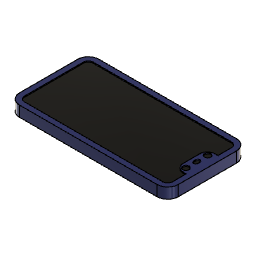
Telefono v5 (Autodesk Fusion 360 design; units mm, degrees)
Autodesk Fusion 360 part; units mm, degrees
sketch "Sketch1" plane through (0, 0, 0) normal (0, 0, 1) x (1, 0, 0)
  line L0 (75, 37.5) -> (-75, 37.5)
  line L1 (-75, 37.5) -> (-75, -37.5)
  line L2 (-75, -37.5) -> (75, -37.5)
  line L3 (75, -37.5) -> (75, 37.5)
  line L4 (75, 37.5) -> (-75, -37.5) construction
  line L5 (-75, 37.5) -> (75, -37.5) construction
  dimension "d1" = 150
  dimension "d2" = 75
  constraint horizontal L0
  constraint perpendicular L0 L1
  constraint parallel L0 L2
  constraint parallel L1 L3
  constraint coincident L4 origin
  constraint coincident L5 origin
  measures "d1" distance of L1.end L2.end
  measures "d2" distance of L0.end L1.end
extrude "Extrude1" add sketch "Sketch1" along normal blind 10
fillet "Fillet1" radius 10 2 edges at (75, -37.5, 5) (75, 37.5, 5)
fillet "Fillet1" radius 10 2 edges at (-75, -37.5, 5) (-75, 37.5, 5)
sketch "Sketch2" plane through (0, 0, 10) normal (0, 0, 1) x (-1, 0, 0)
  arc A0 (65, -37.5) -> (75, -27.5) centre (65, -27.5) ccw
  line L0 (75, -27.5) -> (75, 27.5)
  arc A1 (75, 27.5) -> (65, 37.5) centre (65, 27.5) ccw
  line L1 (65, 37.5) -> (-65, 37.5)
  arc A2 (-65, 37.5) -> (-75, 27.5) centre (-65, 27.5) ccw
  line L2 (-75, 27.5) -> (-75, -27.5)
  arc A3 (-75, -27.5) -> (-65, -37.5) centre (-65, -27.5) ccw
  line L3 (-65, -37.5) -> (65, -37.5)
  line L4 (-70, -32.5) -> (70, -32.5)
  line L5 (70, -32.5) -> (70, 32.5)
  line L6 (70, 32.5) -> (-70, 32.5)
  line L7 (-70, 32.5) -> (-70, -32.5)
  line L8 (-70, -32.5) -> (70, 32.5) construction
  line L9 (70, -32.5) -> (-70, 32.5) construction
  line L10 (60, -15) -> (70, -15)
  line L11 (60, 15) -> (60, -15)
  line L12 (60, -15) -> (80, 15) construction
  line L13 (80, -15) -> (60, 15) construction
  line L14 (70, 15) -> (60, 15)
  line L15 (65, 15) -> (65, -15)
  circle A4 centre (65, 10.2985) radius 3
  circle A5 centre (65, -10.2805) radius 3
  line L16 (63, -3) -> (67, -3)
  line L17 (67, -3) -> (67, 3)
  line L18 (67, 3) -> (63, 3)
  line L19 (63, 3) -> (63, -3)
  line L20 (63, -3) -> (67, 3) construction
  line L21 (67, -3) -> (63, 3) construction
  point P0 (70, 0)
  point P1 (65, 0)
  dimension "d9" = 140
  dimension "d10" = 65
  dimension "d11" = 6
  dimension "d12" = 6
  constraint horizontal L4
  constraint perpendicular L4 L5
  constraint parallel L4 L6
  constraint parallel L5 L7
  constraint coincident L8 origin
  constraint coincident L9 origin
  constraint horizontal L10
  constraint coincident L12 P0
  constraint coincident L13 P0
  constraint midpoint L5 P0
  constraint coincident L5 L10.end
  constraint coincident L5 L14.start
  constraint midpoint L14 L15.start
  constraint midpoint L10 L15.end
  constraint perpendicular L10 L15
  constraint coincident L15 A4.centre
  constraint coincident L15 A5.centre
  constraint horizontal L16
  constraint perpendicular L16 L17
  constraint parallel L16 L18
  constraint parallel L17 L19
  constraint coincident L20 P1
  constraint coincident L21 P1
  constraint midpoint L15 P1
  measures "d9" distance of L5.end L6.end
  measures "d10" distance of L4.end L5.end
  measures "d11" diameter of A4
  measures "d12" diameter of A5
extrude "Extrude3" cut sketch "Sketch2" against normal blind 1 contours L4 L5 L6 L7 L10 L11 L14
extrude "Extrude2" cut sketch "Sketch2" against normal blind 1 contours L15 A5 | L15 A5 | L15 A4 | L15 A4 | L15 L16 L18 L19 | L15 L16 L17 L18
fillet "Fillet2" chord length 10 2 edges at (-60, -15, 9.5) (-60, 15, 9.5)
fillet "Fillet3" radius 2 4 edges at (-63, 3, 9.5) (-67, 3, 9.5) (-67, -3, 9.5) (-63, -3, 9.5)
fillet "Fillet4" chord length 6.5 4 edges at (-70, 32.5, 9.5) (-70, -32.5, 9.5) (70, 32.5, 9.5) (70, -32.5, 9.5)
sketch "Sketch3" plane through (0, 0, 0) normal (0, 1, 0) x (1, 0, 0)
scale "Scale1" factor 0.6 about (65.4038, -32.5, 9) bodies 1
move_body "Move1" bodies 1 to x (0, -1, 0) y (1, 0, 0) z (0, 0, 1) at (-46.6513, 24.489, -29.1736)
move_body "Move2" bodies 1 to x (1, 0, 0) y (0, 1, 0) z (0, 0, 1) at (62.0511, 1.1598, 0)
move_body "Align1" bodies 1 to x (1, 0, 0) y (0, 1, 0) z (0, 0, 1) at (-2.3999, 0.5127, 20.1736)
move_body "Move3" bodies 1 to x (0, -1, 0) y (1, 0, 0) z (0, 0, 1) at (22.5, -67.5, 0)
move_body "Move4" bodies 1 to x (1, 0, 0) y (0, 1, 0) z (0, 0, 1) at (-22.5, 67.5, 5.4)
